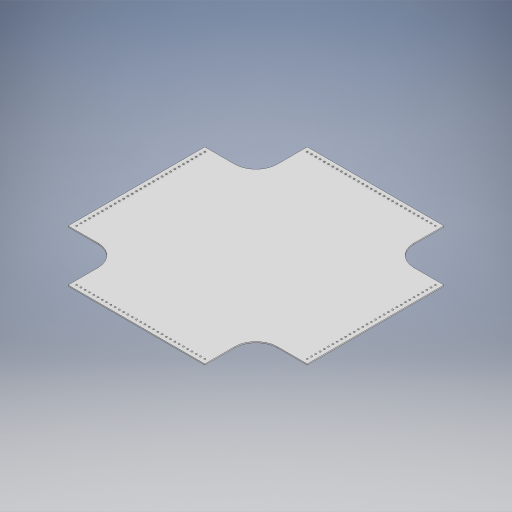
# Autodesk Inventor part: 2024-100-006-Electrical-Plate
Saved by Autodesk Inventor 2024.2 (Build 282272000, 272)
## iProperties
Created: 2024-02-07
Part Number: 2024-100-006-Electrical-Plate
Material: Polycarbonate, Clear
Document SubType Name: Modeling
Designer: rohan
Density: 1.2 g/cm^3
Appearance: No Tint
Author: rohan
Autodesk Inventor part; units mm, degrees
ref_plane "YZ Plane" through (0, 0, 0) normal (1, 0, 0) x (0, 1, 0)
ref_plane "XZ Plane" through (0, 0, 0) normal (0, 1, 0) x (-1, 0, 0)
ref_plane "XY Plane" through (0, 0, 0) normal (0, 0, 1) x (1, 0, 0)
sketch "Sketch1" plane through (0, 0, 0) normal (0, 1, 0) x (-1, 0, 0)
  line L0 (355.6, 355.6) -> (-355.6, 355.6)
  line L1 (-355.6, 355.6) -> (-355.6, -355.6)
  line L2 (-355.6, -355.6) -> (355.6, -355.6)
  line L3 (355.6, -355.6) -> (355.6, 355.6)
  line L4 (355.6, 355.6) -> (-355.6, -355.6) construction
  line L5 (-355.6, 355.6) -> (355.6, -355.6) construction
  point P0 (0, 0)
  dimension "d0" = 711.2
  dimension "d1" = 711.2
  constraints: 12 end point, 2 midpoint, 2 parallel, 1 horizontal, 1 perpendicular
  measures "d0" distance of L2.end L1.end
  measures "d1" distance of L1.end L0.end
extrude "Extrusion1" add sketch "Sketch1" along normal blind 3.175
sketch "Sketch2" plane through (0, 3.175, 0) normal (0, 1, 0) x (1, 0, 0)
  line L0 (355.6, 355.6) -> (-355.6, 355.6) projected
  line L1 (-355.6, 355.6) -> (-203.2, 355.6)
  line L2 (-203.2, 355.6) -> (-203.2, 203.2)
  line L3 (-203.2, 203.2) -> (-355.6, 203.2)
  line L4 (-355.6, 203.2) -> (-355.6, 355.6)
  line L5 (355.6, 355.6) -> (203.2, 355.6)
  line L6 (203.2, 355.6) -> (203.2, 203.2)
  line L7 (203.2, 203.2) -> (355.6, 203.2)
  line L8 (355.6, 203.2) -> (355.6, 355.6)
  line L9 (-355.6, -354.2456) -> (-203.2, -354.2456)
  line L10 (-355.6, -201.8456) -> (-355.6, -354.2456)
  line L11 (355.6, -354.2456) -> (203.2, -354.2456)
  line L12 (355.6, -201.8456) -> (355.6, -354.2456)
  line L13 (355.6, -355.6) -> (355.6, 355.6) projected
  line L14 (355.6, 355.6) -> (-355.6, 355.6) projected
  line L15 (-355.6, 355.6) -> (-355.6, -355.6) projected
  line L16 (-355.6, -355.6) -> (355.6, -355.6) projected
  line L17 (-355.6, -355.6) -> (-203.2, -355.6)
  line L18 (-203.2, -355.6) -> (-203.2, -203.2)
  line L19 (-203.2, -203.2) -> (-355.6, -203.2)
  line L20 (-355.6, -203.2) -> (-355.6, -355.6)
  line L21 (355.6, -355.6) -> (203.2, -355.6)
  line L22 (203.2, -355.6) -> (203.2, -203.2)
  line L23 (203.2, -203.2) -> (355.6, -203.2)
  line L24 (355.6, -203.2) -> (355.6, -355.6)
  point P0 (0, 0)
  dimension "d4" = 152.4
  dimension "d5" = 152.4
  dimension "d6" = 152.4
  dimension "d7" = 152.4
  dimension "d12" = 152.4
  dimension "d13" = 152.4
  dimension "d14" = 152.4
  dimension "d15" = 152.4
  constraints: 40 end point, 8 parallel, 6 horizontal, 4 perpendicular, 3 point on line
  measures "d4" distance of L2.end L3.end
  measures "d5" distance of L1.end L2.end
  measures "d6" distance of L7.end L6.end
  measures "d7" distance of L6.end L5.end
  measures "d12" distance of L19.end L18.end
  measures "d13" distance of L18.end L17.end
  measures "d14" distance of L22.end L23.end
  measures "d15" distance of L21.end L22.end
extrude "Extrusion2" cut sketch "Sketch2" against normal blind 47.625 contours L8 L7 L6 L0 | L2 L3 L4 L0 | L12 L11 L22 L23 | L13 L16 L22 L11 | L19 L18 L9 L10 | L9 L18 L16 L15
fillet "Fillet1" radius 63.5 4 edges at (-203.2, 1.5875, 203.2) (203.2, 1.5875, 203.2) (203.2, 1.5875, -203.2) (-203.2, 1.5875, -203.2)
sketch "Sketch3" plane through (0, 3.175, 0) normal (0, 1, 0) x (1, 0, 0)
  circle A0 centre (190.5, 342.9) radius 2.4892
  line L0 (203.2, 266.7) -> (203.2, 355.6) projected
  line L1 (203.2, 355.6) -> (-203.2, 355.6) projected
  point P0 (0, 0)
  dimension "d19" = 4.9784
  dimension "d20" = 12.7
  dimension "d21" = 12.7
  constraints: 1 centre point
  measures "d19" diameter of A0
  measures "d20" distance from line of L0 A0.centre
  measures "d21" distance from line of L1 A0.centre
extrude "Extrusion3" cut sketch "Sketch3" against normal blind 12.7
pattern_linear "Rectangular Pattern1" count 31 spacing 12.7 along (-1, 0, 0) of "Extrusion3"
sketch "Sketch4" plane through (0, 3.175, 0) normal (0, 1, 0) x (1, 0, 0)
  circle A0 centre (-342.9, 190.5) radius 2.4892
  line L0 (-355.6, 203.2) -> (-355.6, -203.2) projected
  line L1 (-266.7, 203.2) -> (-355.6, 203.2) projected
  point P0 (0, 0)
  dimension "d27" = 4.9784
  dimension "d28" = 12.7
  dimension "d29" = 12.7
  constraints: 1 centre point
  measures "d27" diameter of A0
  measures "d28" distance from line of A0.centre L0
  measures "d29" distance from line of L1 A0.centre
extrude "Extrusion4" cut sketch "Sketch4" against normal blind 15.875
pattern_linear "Rectangular Pattern2" count 31 spacing 12.7 along (0, 0, 1) of "Extrusion4"
sketch "Sketch5" plane through (0, 3.175, 0) normal (0, 1, 0) x (1, 0, 0)
  circle A0 centre (-190.5, -342.9) radius 2.4892
  line L0 (-203.2, -355.6) -> (203.2, -355.6) projected
  line L1 (-203.2, -266.7) -> (-203.2, -355.6) projected
  point P0 (0, 0)
  dimension "d35" = 4.9784
  dimension "d37" = 12.7
  dimension "d66" = 12.7
  constraints: 1 centre point
  measures "d35" diameter of A0
  measures "d37" distance from line of L1 A0.centre
  measures "d66" distance from line of L0 A0.centre
extrude "Extrusion5" cut sketch "Sketch5" against normal blind 11.1125
pattern_linear "Rectangular Pattern3" count 31 spacing 12.7 along (1, 0, 0) of "Extrusion5"
sketch "Sketch6" plane through (0, 3.175, 0) normal (0, 1, 0) x (1, 0, 0)
  circle A0 centre (342.9, -190.5) radius 2.4892
  line L0 (355.6, -203.2) -> (355.6, 203.2) projected
  line L1 (266.7, -203.2) -> (355.6, -203.2) projected
  point P0 (0, 0)
  dimension "d43" = 4.9784
  dimension "d45" = 12.7
  dimension "d67" = 12.7
  constraints: 1 centre point
  measures "d43" diameter of A0
  measures "d45" distance from line of L1 A0.centre
  measures "d67" distance from line of A0.centre L0
extrude "Extrusion6" cut sketch "Sketch6" against normal blind 19.05
pattern_linear "Rectangular Pattern4" count 31 spacing 12.7 along (0, 0, -1) of "Extrusion6"
body "Solid1"
